enz metal 1_v6 (Autodesk Fusion 360 design; units mm, degrees)
Autodesk Fusion 360 part; units mm, degrees
sketch "base" plane through (0, 0, 0) normal (0, 0, 1) x (1, 0, 0)
  circle A0 centre (-22.4, 0.0874) radius 7.15
  circle A1 centre (0, 0) radius 32.75
  circle A2 centre (0, 0) radius 7.15
  circle A3 centre (-15.9191, -15.7337) radius 7.15
  circle A4 centre (-0.1492, -22.3382) radius 7.15
  circle A5 centre (15.672, -15.8573) radius 7.15
  circle A6 centre (22.2765, -0.0874) radius 7.15
  circle A7 centre (15.7956, 15.7337) radius 7.15
  circle A8 centre (0.0256, 22.3382) radius 7.15
  circle A9 centre (-15.7955, 15.8573) radius 7.15
  point P0 (-22.4, 0.0874)
  point P1 (-0.0618, 0)
  dimension "d54" = 14.3
  dimension "d67" = 22.4
  dimension "d68" = 14.3
  dimension "d80" = 360
  dimension "d82" = 65.5
  constraint coincident A1.centre A2.centre
  constraint coincident P0 A0.centre
  measures "d54" diameter of A2
  measures "d67" horizontal distance of P0 A1.centre
  measures "d68" diameter of A0
  measures "d82" diameter of A1
extrude "seat" add sketch "base" along normal blind 2 from surface at 36 makes body 1
sketch "rim" plane through (0, 0, 0) normal (0, 1, 0) x (1, 0, 0)
  line L0 (32.75, -37.2) -> (32.75, -49.2)
  line L1 (32.75, -37.2) -> (31.0508, -37.2)
  line L2 (31.0508, -37.2) -> (31.0508, -49.2)
  line L3 (31.0508, -49.2) -> (32.75, -49.2)
  line L4 (32.75, -49.2) -> (37.1882, -52.2)
  line L5 (31.0508, -49.2) -> (35.4891, -52.2)
  line L6 (35.4891, -52.2) -> (37.1882, -52.2)
  point P0 (32.75, -37.2)
  point P1 (-0.0618, 0)
  point P2 (-0.1492, 0)
  dimension "d26" = 37.2
  dimension "d27" = 32.75
  dimension "d29" = 12
  dimension "d35" = 3
  dimension "d63" = 37.25
  dimension "d89" = 12
  dimension "d91" = 31.2
  constraint coincident P0 L0.start
  constraint perpendicular L0 L1
  constraint perpendicular L1 L2
  constraint parallel L1 L3
  constraint equal L4 L5
  constraint parallel L4 L5
  constraint horizontal L6
  measures "d26" vertical distance of origin L0.start
  measures "d27" horizontal distance of P0 origin
  measures "d29" distance of P0 L0.end
  measures "d35" vertical distance of L0.end L4.end
  measures "d63" horizontal distance of L4.end P1
  measures "d89" distance of L1.end L2.end
  measures "d91" distance of L2 P2
revolve "Revolve2" add sketch "rim" angle 360 about axis through (0, 0, 1.75) along (0, 0, 1) bodies 1
sketch "washer mold" plane through (0, 0, 0) normal (0, 0, 1) x (1, 0, 0)
  circle A0 centre (100, 0) radius 19.375
  circle A1 centre (100, 0) radius 16.375
  circle A2 centre (100, 0) radius 15.625
  circle A3 centre (100, 0) radius 18.625
  point P0 (100, 0)
  dimension "d85" = 37.25
  dimension "d86" = 32.75
  dimension "d87" = 38.75
  dimension "d88" = 31.25
  constraint concentric A1 A3
  constraint concentric A2 A3
  constraint concentric A0 A2
  measures "d85" diameter of A3
  measures "d86" diameter of A1
  measures "d87" diameter of A0
  measures "d88" diameter of A2
extrude "Extrude10" add sketch "washer mold" along normal blind 2 separate body contours A3 makes body 2
extrude "Extrude11" add sketch "washer mold" along normal blind 5 bodies 2
chamfer "Chamfer1" distance 2 angle 45 1 edges at (-28.9496, -11.2285, 38) on bodies 1
fillet "Fillet1" radius 0.2 1 edges at (-28.9496, -11.2285, 49.2) on bodies 1
equation "submergedTubeHeight = 36 mm"
equation "capHeightAndOverhead = 12 mm"
equation "tubHoleDiameter = 14.3 mm"
equation "largeRimOutsideDiameter = 74.5 mm"
equation "baseRimOutsideDiameter = largeRimOutsideDiameter - 9 mm"
equation "generalThickness = 2 mm"
equation "tubeWallThickness = 1.2 mm"
equation "d26 = submergedTubeHeight + tubeWallThickness"
equation "d27 = baseRimOutsideDiameter / 2"
equation "d29 = capHeightAndOverhead"
equation "d42 = submergedTubeHeight + tubeBottomThickness - generalThickness"
equation "d43 = generalThickness"
equation "d54 = tubHoleDiameter"
equation "d63 = largeRimOutsideDiameter / 2"
equation "tubeBottomThickness = 2 mm"
equation "d68 = tubHoleDiameter"
equation "d85 = largeRimOutsideDiameter / 2"
equation "d86 = ( baseRimOutsideDiameter / 2 mm ) * 1 mm"
equation "d87 = largeRimOutsideDiameter / 2 + 1.5 mm"
equation "d88 = baseRimOutsideDiameter / 2 - 1.5 mm"
equation "d80 = 360.0 °"
equation "d82 = baseRimOutsideDiameter"
equation "d91 = baseRimInteriorDiameter / 2"
equation "baseRimInteriorDiameter = 62.4 mm"
named bodies: "holder", "washerMold"
